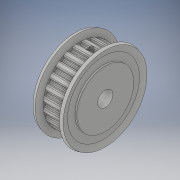
# Autodesk Inventor part: C-ATP24XL037-A-P8
Saved by Autodesk Inventor 2019 (Build 230136000, 136)
## iProperties
Created: 2023-01-11
Part Number: C-ATP24XL037-A-P8
Material: Generic
Catalog Web Link: www.cadenas.de
Description: C-ATP__XL025, C-ATP__XL031, C-ATP__ XL037, C-ATP__XL050-Economy Timing Pulleys XL Type
Vendor: MISUMI
Document SubType Name: Modeling
Designer: psAdmin
Manufacturer: MISUMI
Mass: 17.241 g
Surface Area: 69.8736 cm^2
Volume: 17.241 cm^3
Density: 1 g/cm^3
Appearance: PSOLRGB-175-175-175
Category: PARTsolutions
Company: MISUMI
Title: C-ATP24XL037-A-P8
Author: Cadenas PARTsolutions
Comments: Economy Timing Pulleys XL Type
PSOL_IDENT_0: {$CADENAS_DATA/23d-libs/misumi/metric/51_timing_pulleys/c_atp_xl.prj},239 {VTYP=3D},{NB=C-ATP24XL037
PSOL_IDENT_1: -A-P8},{LINA=C-ATP24XL037-A-P8},{NN=C-ATP__XL025, C-ATP__XL031, C-ATP__ XL037, C-ATP__XL050},{DATE=2
PSOL_IDENT_2: 2.09.2022 05:17:01},{GEOMDATE=17.04.2021 17:32:28},{VERSION=},{LINEID=110},{WBVAR=TNW,PS,SBS,DD},{WB
PSOL_IDENT_3: NUMERIC=DD}  {NB=C-ATP24XL037-A-P8},{LINA=C-ATP24XL037-A-P8},{KT=DUMMY},{PN=C-ATP24XL037-A-P8},{TYPE=
PSOL_IDENT_4: C-ATP},{MATP=},{MATPALG= 'A2017','Aluminum Alloy 2000 series','S45C','1045 Carbon Steel Equivalent','
PSOL_IDENT_5: SUS304','SUS304' },{ST=},{STALG=},{NT=24},{TNW=XL037},{TNWALG= 'XL037' },{BW=9.5mm (3/8inch)},{PS=A}
PSOL_IDENT_6: ,{PSALG= 'A' },{SBS=P},{SBSALG= 'P','Round Hole + Tap' },{DD=8.00},{DDALG=8,10},{DDHA=[8:12/1],12.7,
PSOL_IDENT_7: [13:26/1]},{DDPA=8,10},{DDNA=},{DDNK=10},{DDCA=[10,12,15,16,18,19,20]},{DDVA=[8:12/1],12.7,[13:24/1]
PSOL_IDENT_8: },{DDY=[8:24/1]},{DDWB=[8:22/1]},{DDHB=},{DDPB=},{DDNB=8,14,15},{DDCB=},{DDVFB=},{Z=0},{ZALG=[0]},{Z
PSOL_IDENT_9: MIN=10.000},{ZAMAX=26.000},{ZBMAX=0.000},{DDZ=8.000},{J=0.0},{JALG=[0]},{JMIN=2.000},{JMAX=14.0},{JP
PSOL_IDENT_10: N=},{Q=0},{QALG=[0]},{QRMIN=10.000},{QRMAX=26},{WBQMIN=12.000},{R=0},{RALG=[0]},{WBRMAX=-2.000},{S=0
PSOL_IDENT_11: .0},{SALG=[0]},{SMAX=8},{T=0.0},{TALG=[0]},{TMAX=8},{SBSPN=-P8},{A=11.0},{W=16.0},{L=0},{PD=38.81},{
PSOL_IDENT_12: OD=38.30},{D=0},{DALG=26.000},{DE=30},{F=45},{E=30},{TT=1.6},{BBK=0.000},{TTK=0.0},{ALT1=},{ALT1ALG=
PSOL_IDENT_13: '','w/o KC90 (Set Screw Angle)','KC90','with KC90 (Set Screw Angle)' },{ANG=120.000},{ALT1PN=},{ALT
PSOL_IDENT_14: 2=},{ALT2ALG= '','w/o Side Tapped Hole','QTC','with QTC (3 Places Side Tapped Hole)' },{M=},{MALG= '
PSOL_IDENT_15: N/A' },{MFTALG= 'N/A' },{MSALG= 'N/A' },{M3D=0.000},{KDML=0.000},{ML=0.000},{MUL=0.000},{PITCH=0.000
PSOL_IDENT_16: },{QSC=0.0},{QSCALG=0},{QFC=0.0},{QFCALG=0},{QTC=0.0},{QTCALG=0},{QPCDMIN=0.000},{QPCDMINALG=0.000},
PSOL_IDENT_17: {QPCDMAX=26.000},{ALT2PN=},{TAP=0.000},{ALT3=},{ALT3ALG= '','w/o Side Through Hole','KTC','with KTC
PSOL_IDENT_18: (3 Places Side Through Hole)' },{K=0.0},{KALG=0},{KMIN=4.000},{KFTMAX=7.000},{KSMAX=7.000},{KSC=0.0}
PSOL_IDENT_19: ,{KSCALG=0},{KFC=0.0},{KFCALG=0},{KTC=0.0},{KTCALG=0},{KSCMIN=12.000},{KPCDMIN=12.000},{KPCDMAX=26.0
PSOL_IDENT_20: 00},{ALT3PN=},{ALT4=},{ALT4ALG= '','w/o Side Counterbored','ZTC','with ZTC (3 Places Side Counterbor
PSOL_IDENT_21: ed)' },{ALT4MIN=18.500},{ALT4MAX=19.500},{ZM=},{ZMALG= 'N/A' },{ZMFTALG= 'N/A' },{ZMSALG= 'N/A' },{Z
PSOL_IDENT_22: MDD1=0.0},{ZMDD2=0.0},{ZMHH=0.0},{ZSC=0.0},{ZSCALG=[0]},{ZFC=0.0},{ZFCALG=[0]},{ZTC=0.0},{ZTCALG=[0]
PSOL_IDENT_23: },{ZPCDMIN=0.000},{ZPCDMINALG=0.000},{ZPCDMAX=26.000},{ALT4PN=},{ALT5=},{ALT5ALG= '','w/o Flange not
PSOL_IDENT_24: Attached','NFC','with NFC (Flange not Attached)' },{ALT5PN=},{ALT6=},{ALT6ALG= '','w/o Flange Attac
PSOL_IDENT_25: hed on One Side Only','RFC','with RFC (Flange Attached on The Boss Side Only)','LFC','with LFC (Flan
PSOL_IDENT_26: ge Attached on The Opposite Side Only)' },{ALT6PN=},{ALT7=},{ALT7ALG= '','w/o FC (Flange Cut)','FC','
PSOL_IDENT_27: with FC (Flange Cut)' },{FC=0.0},{FCALG=0},{FCMIN=39.5},{FCMAX=43.0},{ALT7PN=},{ALT8=},{ALT8ALG= '','
PSOL_IDENT_28: Not applicable' },{ALT8ALGALG=26.000},{ALT8DD2=0.000},{ALT8MM=0.000},{ALT8NN=0.000},{QC=0.000},{KC=0
PSOL_IDENT_29: .000},{ZC=0.000},{SRG=0.0},{SRGALG=[0]},{SRGMAX=0.000},{DD2=0.0},{MM=0.00},{NN=0.00},{ALT8PN=},{ALT9=
PSOL_IDENT_30: },{ALT9ALG= '','w/o BTC (Taper for Bearing Holder)','BTC','with BTC (Taper for Bearing Holder)' },{B
PSOL_IDENT_31: TC9=9.000},{TL9=1.000},{BTC=0},{BTCALG=[0]},{TL=0.0},{TLALG=0},{TLMIN=1.000},{TLMAX=-16.500},{BTCL=0
PSOL_IDENT_32: },{BTCD=0},{ALT9PN=},{WLBCTL=16.000},{ALT10=},{ALT10ALG= '','w/o TPC (Tapped Hole Dimension)','TPC','
PSOL_IDENT_33: with TPC (Tapped Hole Dimension)' },{TPC=},{TPCALG= 'N/A' },{TPCM=4.000},{ALT10PN=},{ALT11=},{ALT11A
PSOL_IDENT_34: LG= '','Not applicable' },{BC=0.0},{BCALG=0},{BCMIN=7},{BCMAX=-16.5},{M1WBC=8},{ALT11PN=},{KTT=15.15
PSOL_IDENT_35: },{ALT12=},{ALT12ALG= '','w/o SLH (Set Screw Length)','SLH','with SLH (Set Screw Length)' },{SLH=0},
PSOL_IDENT_36: {SLHALG=[0]},{ALT12PN=},{AC=M4x3},{M1=4.000},{M1L=3.000},{KEYA=1.000},{KEYB=0.000},{KEYM=1.000}
NB: C-ATP24XL037-A-P8
NN: C-ATP__XL025, C-ATP__XL031, C-ATP__ XL037, C-ATP__XL050
NT: 24
NBSYN: $PN.
LINA: C-ATP24XL037-A-P8
CATALOG: Misumi
PN: C-ATP24XL037-A-P8
TNW: XL037
PS: A
SBS: Round Hole + Tap
DD: 8
PD: 38.81
OD: 38.3
D: 0
F: 45
E: 30
SUPPLIER: MISUMI
ARTICLENO: C-ATP24XL037-A-P8
BOMINFO: C-ATP24XL037-A-P8
CREATOR: CADENAS GmbH
Autodesk Inventor part; units mm, degrees
sketch "_____2" plane through (0, 0, 0) normal (0, 0, 1) x (1, 0, 0)
  line L0 (16, 0) -> (0, 0)
  line L1 (0, 0) -> (0, 15)
  line L2 (0, 15) -> (0.9, 15)
  line L3 (0.9, 15) -> (0.9, 18.9394)
  line L4 (0.9, 18.9394) -> (0.0569, 22.0859)
  line L5 (0.0569, 22.0859) -> (1.6024, 22.5)
  line L6 (1.6024, 22.5) -> (2.5, 19.15)
  line L7 (2.5, 19.15) -> (13.5, 19.15)
  line L8 (13.5, 19.15) -> (14.3976, 22.5)
  line L9 (14.3976, 22.5) -> (15.9431, 22.0859)
  line L10 (15.9431, 22.0859) -> (15.1, 18.9394)
  line L11 (15.1, 18.9394) -> (15.1, 15)
  line L12 (15.1, 15) -> (16, 15)
  line L13 (16, 15) -> (16, 0)
  line L14 (16, 0) -> (0, 0)
  constraints: 30 end point
revolve "Revolution1" add sketch "_____2" angle 360 about axis through (16, 0, 0) along (1, 0, 0)
sketch "Sketch2" plane through (16, 0, 0) normal (1, 0, 0) x (0, 0, -1)
  point P0 (0, 0)
hole "Hole1" at (16, 0, 0) direction (-1, 0, 0) diameter 8 depth 16
sketch "_____6" plane through (2.5, 0, 0) normal (1, 0, 0) x (0, 0, -1)
  arc A0 (-19.239, 2.5329) -> (-19.239, -2.5329) centre (0, 0) ccw
  arc A1 (-19.239, -2.5329) -> (-17.9279, -7.426) centre (0, 0) ccw
  arc A2 (-17.9279, -7.426) -> (-15.395, -11.813) centre (0, 0) ccw
  arc A3 (-15.395, -11.813) -> (-11.813, -15.395) centre (0, 0) ccw
  arc A4 (-11.813, -15.395) -> (-7.426, -17.9279) centre (0, 0) ccw
  arc A5 (-7.426, -17.9279) -> (-2.5329, -19.239) centre (0, 0) ccw
  arc A6 (-2.5329, -19.239) -> (2.5329, -19.239) centre (0, 0) ccw
  arc A7 (2.5329, -19.239) -> (7.426, -17.9279) centre (0, 0) ccw
  arc A8 (7.426, -17.9279) -> (11.813, -15.395) centre (0, 0) ccw
  arc A9 (11.813, -15.395) -> (15.395, -11.813) centre (0, 0) ccw
  arc A10 (15.395, -11.813) -> (17.9279, -7.426) centre (0, 0) ccw
  arc A11 (17.9279, -7.426) -> (19.239, -2.5329) centre (0, 0) ccw
  arc A12 (19.239, -2.5329) -> (19.239, 2.5329) centre (0, 0) ccw
  arc A13 (19.239, 2.5329) -> (17.9279, 7.426) centre (0, 0) ccw
  arc A14 (17.9279, 7.426) -> (15.395, 11.813) centre (0, 0) ccw
  arc A15 (15.395, 11.813) -> (11.813, 15.395) centre (0, 0) ccw
  arc A16 (11.813, 15.395) -> (7.426, 17.9279) centre (0, 0) ccw
  arc A17 (7.426, 17.9279) -> (2.5329, 19.239) centre (0, 0) ccw
  arc A18 (2.5329, 19.239) -> (-2.5329, 19.239) centre (0, 0) ccw
  arc A19 (-2.5329, 19.239) -> (-7.426, 17.9279) centre (0, 0) ccw
  arc A20 (-7.426, 17.9279) -> (-11.813, 15.395) centre (0, 0) ccw
  arc A21 (-11.813, 15.395) -> (-15.395, 11.813) centre (0, 0) ccw
  arc A22 (-15.395, 11.813) -> (-17.9279, 7.426) centre (0, 0) ccw
  arc A23 (-17.9279, 7.426) -> (-19.239, 2.5329) centre (0, 0) ccw
  arc A24 (-18.7244, -1.0947) -> (-19.0742, -1.7017) centre (-18.4667, -1.6475) ccw
  arc A25 (-19.0742, -1.7017) -> (-18.9862, -2.4996) centre (0, 0) ccw
  arc A26 (-18.9862, -2.4996) -> (-18.8647, -3.293) centre (0, 0) ccw
  arc A27 (-18.8647, -3.293) -> (-18.3698, -3.7889) centre (-18.2638, -3.1881) ccw
  line L0 (-18.3698, -3.7889) -> (-17.6918, -3.9084)
  arc A28 (-17.2064, -4.3593) -> (-17.6918, -3.9084) centre (-17.7977, -4.5091) ccw
  arc A29 (-17.2064, -4.3593) -> (-17.0808, -4.8279) centre (0, 0) ccw
  arc A30 (-17.2757, -5.4611) -> (-17.0808, -4.8279) centre (-17.6678, -4.9938) ccw
  line L1 (-17.2757, -5.4611) -> (-17.8031, -5.9036)
  arc A31 (-17.8031, -5.9036) -> (-17.9839, -6.5805) centre (-17.411, -6.3709) ccw
  arc A32 (-17.9839, -6.5805) -> (-17.6923, -7.3284) centre (0, 0) ccw
  arc A33 (-17.6923, -7.3284) -> (-17.3696, -8.0634) centre (0, 0) ccw
  arc A34 (-17.3696, -8.0634) -> (-16.7632, -8.4142) centre (-16.8164, -7.8065) ccw
  line L2 (-16.7632, -8.4142) -> (-16.0773, -8.3542)
  arc A35 (-15.4918, -8.6641) -> (-16.0773, -8.3542) centre (-16.0242, -8.9619) ccw
  arc A36 (-15.4918, -8.6641) -> (-15.2492, -9.0842) centre (0, 0) ccw
  arc A37 (-15.2736, -9.7463) -> (-15.2492, -9.0842) centre (-15.7733, -9.3964) ccw
  line L3 (-15.2736, -9.7463) -> (-15.6685, -10.3103)
  arc A38 (-15.6685, -10.3103) -> (-15.6679, -11.0109) centre (-15.1688, -10.6601) ccw
  arc A39 (-15.6679, -11.0109) -> (-15.1927, -11.6578) centre (0, 0) ccw
  arc A40 (-15.1927, -11.6578) -> (-14.6908, -12.2842) centre (0, 0) ccw
  arc A41 (-14.6908, -12.2842) -> (-14.0142, -12.4661) centre (-14.2229, -11.8929) ccw
  line L4 (-14.0142, -12.4661) -> (-13.3673, -12.2307)
  arc A42 (-12.7215, -12.3785) -> (-13.3673, -12.2307) centre (-13.1587, -12.8039) ccw
  arc A43 (-12.7215, -12.3785) -> (-12.3785, -12.7215) centre (0, 0) ccw
  arc A44 (-12.2307, -13.3673) -> (-12.3785, -12.7215) centre (-12.8039, -13.1587) ccw
  line L5 (-12.2307, -13.3673) -> (-12.4661, -14.0142)
  arc A45 (-12.4661, -14.0142) -> (-12.2842, -14.6908) centre (-11.8929, -14.2229) ccw
  arc A46 (-12.2842, -14.6908) -> (-11.6578, -15.1927) centre (0, 0) ccw
  arc A47 (-11.6578, -15.1927) -> (-11.0109, -15.6679) centre (0, 0) ccw
  arc A48 (-11.0109, -15.6679) -> (-10.3103, -15.6685) centre (-10.6601, -15.1688) ccw
  line L6 (-10.3103, -15.6685) -> (-9.7463, -15.2736)
  arc A49 (-9.0842, -15.2492) -> (-9.7463, -15.2736) centre (-9.3964, -15.7733) ccw
  arc A50 (-9.0842, -15.2492) -> (-8.6641, -15.4918) centre (0, 0) ccw
  arc A51 (-8.3542, -16.0773) -> (-8.6641, -15.4918) centre (-8.9619, -16.0242) ccw
  line L7 (-8.3542, -16.0773) -> (-8.4142, -16.7632)
  arc A52 (-8.4142, -16.7632) -> (-8.0634, -17.3696) centre (-7.8065, -16.8164) ccw
  arc A53 (-8.0634, -17.3696) -> (-7.3284, -17.6923) centre (0, 0) ccw
  arc A54 (-7.3284, -17.6923) -> (-6.5805, -17.9839) centre (0, 0) ccw
  arc A55 (-6.5805, -17.9839) -> (-5.9036, -17.8031) centre (-6.3709, -17.411) ccw
  line L8 (-5.9036, -17.8031) -> (-5.4611, -17.2757)
  arc A56 (-4.8279, -17.0808) -> (-5.4611, -17.2757) centre (-4.9938, -17.6678) ccw
  arc A57 (-4.8279, -17.0808) -> (-4.3593, -17.2064) centre (0, 0) ccw
  arc A58 (-3.9084, -17.6918) -> (-4.3593, -17.2064) centre (-4.5091, -17.7977) ccw
  line L9 (-3.9084, -17.6918) -> (-3.7889, -18.3698)
  arc A59 (-3.7889, -18.3698) -> (-3.293, -18.8647) centre (-3.1881, -18.2638) ccw
  arc A60 (-3.293, -18.8647) -> (-2.4996, -18.9862) centre (0, 0) ccw
  arc A61 (-2.4996, -18.9862) -> (-1.7017, -19.0742) centre (0, 0) ccw
  arc A62 (-1.7017, -19.0742) -> (-1.0947, -18.7244) centre (-1.6475, -18.4667) ccw
  line L10 (-1.0947, -18.7244) -> (-0.8037, -18.1005)
  arc A63 (-0.2426, -17.7483) -> (-0.8037, -18.1005) centre (-0.2509, -18.3583) ccw
  arc A64 (-0.2426, -17.7483) -> (0.2426, -17.7483) centre (0, 0) ccw
  arc A65 (0.8037, -18.1005) -> (0.2426, -17.7483) centre (0.2509, -18.3583) ccw
  line L11 (0.8037, -18.1005) -> (1.0947, -18.7244)
  arc A66 (1.0947, -18.7244) -> (1.7017, -19.0742) centre (1.6475, -18.4667) ccw
  arc A67 (1.7017, -19.0742) -> (2.4996, -18.9862) centre (0, 0) ccw
  arc A68 (2.4996, -18.9862) -> (3.293, -18.8647) centre (0, 0) ccw
  arc A69 (3.293, -18.8647) -> (3.7889, -18.3698) centre (3.1881, -18.2638) ccw
  line L12 (3.7889, -18.3698) -> (3.9084, -17.6918)
  arc A70 (4.3593, -17.2064) -> (3.9084, -17.6918) centre (4.5091, -17.7977) ccw
  arc A71 (4.3593, -17.2064) -> (4.8279, -17.0808) centre (0, 0) ccw
  arc A72 (5.4611, -17.2757) -> (4.8279, -17.0808) centre (4.9938, -17.6678) ccw
  line L13 (5.4611, -17.2757) -> (5.9036, -17.8031)
  arc A73 (5.9036, -17.8031) -> (6.5805, -17.9839) centre (6.3709, -17.411) ccw
  arc A74 (6.5805, -17.9839) -> (7.3284, -17.6923) centre (0, 0) ccw
  arc A75 (7.3284, -17.6923) -> (8.0634, -17.3696) centre (0, 0) ccw
  arc A76 (8.0634, -17.3696) -> (8.4142, -16.7632) centre (7.8065, -16.8164) ccw
  line L14 (8.4142, -16.7632) -> (8.3542, -16.0773)
  arc A77 (8.6641, -15.4918) -> (8.3542, -16.0773) centre (8.9619, -16.0242) ccw
  arc A78 (8.6641, -15.4918) -> (9.0842, -15.2492) centre (0, 0) ccw
  arc A79 (9.7463, -15.2736) -> (9.0842, -15.2492) centre (9.3964, -15.7733) ccw
  line L15 (9.7463, -15.2736) -> (10.3103, -15.6685)
  arc A80 (10.3103, -15.6685) -> (11.0109, -15.6679) centre (10.6601, -15.1688) ccw
  arc A81 (11.0109, -15.6679) -> (11.6578, -15.1927) centre (0, 0) ccw
  arc A82 (11.6578, -15.1927) -> (12.2842, -14.6908) centre (0, 0) ccw
  arc A83 (12.2842, -14.6908) -> (12.4661, -14.0142) centre (11.8929, -14.2229) ccw
  line L16 (12.4661, -14.0142) -> (12.2307, -13.3673)
  arc A84 (12.3785, -12.7215) -> (12.2307, -13.3673) centre (12.8039, -13.1587) ccw
  arc A85 (12.3785, -12.7215) -> (12.7215, -12.3785) centre (0, 0) ccw
  arc A86 (13.3673, -12.2307) -> (12.7215, -12.3785) centre (13.1587, -12.8039) ccw
  line L17 (13.3673, -12.2307) -> (14.0142, -12.4661)
  arc A87 (14.0142, -12.4661) -> (14.6908, -12.2842) centre (14.2229, -11.8929) ccw
  arc A88 (14.6908, -12.2842) -> (15.1927, -11.6578) centre (0, 0) ccw
  arc A89 (15.1927, -11.6578) -> (15.6679, -11.0109) centre (0, 0) ccw
  arc A90 (15.6679, -11.0109) -> (15.6685, -10.3103) centre (15.1688, -10.6601) ccw
  line L18 (15.6685, -10.3103) -> (15.2736, -9.7463)
  arc A91 (15.2492, -9.0842) -> (15.2736, -9.7463) centre (15.7733, -9.3964) ccw
  arc A92 (15.2492, -9.0842) -> (15.4918, -8.6641) centre (0, 0) ccw
  arc A93 (16.0773, -8.3542) -> (15.4918, -8.6641) centre (16.0242, -8.9619) ccw
  line L19 (16.0773, -8.3542) -> (16.7632, -8.4142)
  arc A94 (16.7632, -8.4142) -> (17.3696, -8.0634) centre (16.8164, -7.8065) ccw
  arc A95 (17.3696, -8.0634) -> (17.6923, -7.3284) centre (0, 0) ccw
  arc A96 (17.6923, -7.3284) -> (17.9839, -6.5805) centre (0, 0) ccw
  arc A97 (17.9839, -6.5805) -> (17.8031, -5.9036) centre (17.411, -6.3709) ccw
  line L20 (17.8031, -5.9036) -> (17.2757, -5.4611)
  arc A98 (17.0808, -4.8279) -> (17.2757, -5.4611) centre (17.6678, -4.9938) ccw
  arc A99 (17.0808, -4.8279) -> (17.2064, -4.3593) centre (0, 0) ccw
  arc A100 (17.6918, -3.9084) -> (17.2064, -4.3593) centre (17.7977, -4.5091) ccw
  line L21 (17.6918, -3.9084) -> (18.3698, -3.7889)
  arc A101 (18.3698, -3.7889) -> (18.8647, -3.293) centre (18.2638, -3.1881) ccw
  arc A102 (18.8647, -3.293) -> (18.9862, -2.4996) centre (0, 0) ccw
  arc A103 (18.9862, -2.4996) -> (19.0742, -1.7017) centre (0, 0) ccw
  arc A104 (19.0742, -1.7017) -> (18.7244, -1.0947) centre (18.4667, -1.6475) ccw
  line L22 (18.7244, -1.0947) -> (18.1005, -0.8037)
  arc A105 (17.7483, -0.2426) -> (18.1005, -0.8037) centre (18.3583, -0.2509) ccw
  arc A106 (17.7483, -0.2426) -> (17.7483, 0.2426) centre (0, 0) ccw
  arc A107 (18.1005, 0.8037) -> (17.7483, 0.2426) centre (18.3583, 0.2509) ccw
  line L23 (18.1005, 0.8037) -> (18.7244, 1.0947)
  arc A108 (18.7244, 1.0947) -> (19.0742, 1.7017) centre (18.4667, 1.6475) ccw
  arc A109 (19.0742, 1.7017) -> (18.9862, 2.4996) centre (0, 0) ccw
  arc A110 (18.9862, 2.4996) -> (18.8647, 3.293) centre (0, 0) ccw
  arc A111 (18.8647, 3.293) -> (18.3698, 3.7889) centre (18.2638, 3.1881) ccw
  line L24 (18.3698, 3.7889) -> (17.6918, 3.9084)
  arc A112 (17.2064, 4.3593) -> (17.6918, 3.9084) centre (17.7977, 4.5091) ccw
  arc A113 (17.2064, 4.3593) -> (17.0808, 4.8279) centre (0, 0) ccw
  arc A114 (17.2757, 5.4611) -> (17.0808, 4.8279) centre (17.6678, 4.9938) ccw
  line L25 (17.2757, 5.4611) -> (17.8031, 5.9036)
  arc A115 (17.8031, 5.9036) -> (17.9839, 6.5805) centre (17.411, 6.3709) ccw
  arc A116 (17.9839, 6.5805) -> (17.6923, 7.3284) centre (0, 0) ccw
  arc A117 (17.6923, 7.3284) -> (17.3696, 8.0634) centre (0, 0) ccw
  arc A118 (17.3696, 8.0634) -> (16.7632, 8.4142) centre (16.8164, 7.8065) ccw
  line L26 (16.7632, 8.4142) -> (16.0773, 8.3542)
  arc A119 (15.4918, 8.6641) -> (16.0773, 8.3542) centre (16.0242, 8.9619) ccw
  arc A120 (15.4918, 8.6641) -> (15.2492, 9.0842) centre (0, 0) ccw
  arc A121 (15.2736, 9.7463) -> (15.2492, 9.0842) centre (15.7733, 9.3964) ccw
  line L27 (15.2736, 9.7463) -> (15.6685, 10.3103)
  arc A122 (15.6685, 10.3103) -> (15.6679, 11.0109) centre (15.1688, 10.6601) ccw
  arc A123 (15.6679, 11.0109) -> (15.1927, 11.6578) centre (0, 0) ccw
  arc A124 (15.1927, 11.6578) -> (14.6908, 12.2842) centre (0, 0) ccw
  arc A125 (14.6908, 12.2842) -> (14.0142, 12.4661) centre (14.2229, 11.8929) ccw
  line L28 (14.0142, 12.4661) -> (13.3673, 12.2307)
  arc A126 (12.7215, 12.3785) -> (13.3673, 12.2307) centre (13.1587, 12.8039) ccw
  arc A127 (12.7215, 12.3785) -> (12.3785, 12.7215) centre (0, 0) ccw
  arc A128 (12.2307, 13.3673) -> (12.3785, 12.7215) centre (12.8039, 13.1587) ccw
  line L29 (12.2307, 13.3673) -> (12.4661, 14.0142)
  arc A129 (12.4661, 14.0142) -> (12.2842, 14.6908) centre (11.8929, 14.2229) ccw
  arc A130 (12.2842, 14.6908) -> (11.6578, 15.1927) centre (0, 0) ccw
  arc A131 (11.6578, 15.1927) -> (11.0109, 15.6679) centre (0, 0) ccw
  arc A132 (11.0109, 15.6679) -> (10.3103, 15.6685) centre (10.6601, 15.1688) ccw
  line L30 (10.3103, 15.6685) -> (9.7463, 15.2736)
  arc A133 (9.0842, 15.2492) -> (9.7463, 15.2736) centre (9.3964, 15.7733) ccw
  arc A134 (9.0842, 15.2492) -> (8.6641, 15.4918) centre (0, 0) ccw
  arc A135 (8.3542, 16.0773) -> (8.6641, 15.4918) centre (8.9619, 16.0242) ccw
  line L31 (8.3542, 16.0773) -> (8.4142, 16.7632)
  arc A136 (8.4142, 16.7632) -> (8.0634, 17.3696) centre (7.8065, 16.8164) ccw
  arc A137 (8.0634, 17.3696) -> (7.3284, 17.6923) centre (0, 0) ccw
  arc A138 (7.3284, 17.6923) -> (6.5805, 17.9839) centre (0, 0) ccw
  arc A139 (6.5805, 17.9839) -> (5.9036, 17.8031) centre (6.3709, 17.411) ccw
  line L32 (5.9036, 17.8031) -> (5.4611, 17.2757)
  arc A140 (4.8279, 17.0808) -> (5.4611, 17.2757) centre (4.9938, 17.6678) ccw
  arc A141 (4.8279, 17.0808) -> (4.3593, 17.2064) centre (0, 0) ccw
  arc A142 (3.9084, 17.6918) -> (4.3593, 17.2064) centre (4.5091, 17.7977) ccw
  line L33 (3.9084, 17.6918) -> (3.7889, 18.3698)
  arc A143 (3.7889, 18.3698) -> (3.293, 18.8647) centre (3.1881, 18.2638) ccw
  arc A144 (3.293, 18.8647) -> (2.4996, 18.9862) centre (0, 0) ccw
  arc A145 (2.4996, 18.9862) -> (1.7017, 19.0742) centre (0, 0) ccw
  arc A146 (1.7017, 19.0742) -> (1.0947, 18.7244) centre (1.6475, 18.4667) ccw
  line L34 (1.0947, 18.7244) -> (0.8037, 18.1005)
  arc A147 (0.2426, 17.7483) -> (0.8037, 18.1005) centre (0.2509, 18.3583) ccw
  arc A148 (0.2426, 17.7483) -> (-0.2426, 17.7483) centre (0, 0) ccw
  arc A149 (-0.8037, 18.1005) -> (-0.2426, 17.7483) centre (-0.2509, 18.3583) ccw
  line L35 (-0.8037, 18.1005) -> (-1.0947, 18.7244)
  arc A150 (-1.0947, 18.7244) -> (-1.7017, 19.0742) centre (-1.6475, 18.4667) ccw
  arc A151 (-1.7017, 19.0742) -> (-2.4996, 18.9862) centre (0, 0) ccw
  arc A152 (-2.4996, 18.9862) -> (-3.293, 18.8647) centre (0, 0) ccw
  arc A153 (-3.293, 18.8647) -> (-3.7889, 18.3698) centre (-3.1881, 18.2638) ccw
  line L36 (-3.7889, 18.3698) -> (-3.9084, 17.6918)
  arc A154 (-4.3593, 17.2064) -> (-3.9084, 17.6918) centre (-4.5091, 17.7977) ccw
  arc A155 (-4.3593, 17.2064) -> (-4.8279, 17.0808) centre (0, 0) ccw
  arc A156 (-5.4611, 17.2757) -> (-4.8279, 17.0808) centre (-4.9938, 17.6678) ccw
  line L37 (-5.4611, 17.2757) -> (-5.9036, 17.8031)
  arc A157 (-5.9036, 17.8031) -> (-6.5805, 17.9839) centre (-6.3709, 17.411) ccw
  arc A158 (-6.5805, 17.9839) -> (-7.3284, 17.6923) centre (0, 0) ccw
  arc A159 (-7.3284, 17.6923) -> (-8.0634, 17.3696) centre (0, 0) ccw
  arc A160 (-8.0634, 17.3696) -> (-8.4142, 16.7632) centre (-7.8065, 16.8164) ccw
  line L38 (-8.4142, 16.7632) -> (-8.3542, 16.0773)
  arc A161 (-8.6641, 15.4918) -> (-8.3542, 16.0773) centre (-8.9619, 16.0242) ccw
  arc A162 (-8.6641, 15.4918) -> (-9.0842, 15.2492) centre (0, 0) ccw
  arc A163 (-9.7463, 15.2736) -> (-9.0842, 15.2492) centre (-9.3964, 15.7733) ccw
  line L39 (-9.7463, 15.2736) -> (-10.3103, 15.6685)
  arc A164 (-10.3103, 15.6685) -> (-11.0109, 15.6679) centre (-10.6601, 15.1688) ccw
  arc A165 (-11.0109, 15.6679) -> (-11.6578, 15.1927) centre (0, 0) ccw
  arc A166 (-11.6578, 15.1927) -> (-12.2842, 14.6908) centre (0, 0) ccw
  arc A167 (-12.2842, 14.6908) -> (-12.4661, 14.0142) centre (-11.8929, 14.2229) ccw
  line L40 (-12.4661, 14.0142) -> (-12.2307, 13.3673)
  arc A168 (-12.3785, 12.7215) -> (-12.2307, 13.3673) centre (-12.8039, 13.1587) ccw
  arc A169 (-12.3785, 12.7215) -> (-12.7215, 12.3785) centre (0, 0) ccw
  arc A170 (-13.3673, 12.2307) -> (-12.7215, 12.3785) centre (-13.1587, 12.8039) ccw
  line L41 (-13.3673, 12.2307) -> (-14.0142, 12.4661)
  arc A171 (-14.0142, 12.4661) -> (-14.6908, 12.2842) centre (-14.2229, 11.8929) ccw
  arc A172 (-14.6908, 12.2842) -> (-15.1927, 11.6578) centre (0, 0) ccw
  arc A173 (-15.1927, 11.6578) -> (-15.6679, 11.0109) centre (0, 0) ccw
  arc A174 (-15.6679, 11.0109) -> (-15.6685, 10.3103) centre (-15.1688, 10.6601) ccw
  line L42 (-15.6685, 10.3103) -> (-15.2736, 9.7463)
  arc A175 (-15.2492, 9.0842) -> (-15.2736, 9.7463) centre (-15.7733, 9.3964) ccw
  arc A176 (-15.2492, 9.0842) -> (-15.4918, 8.6641) centre (0, 0) ccw
  arc A177 (-16.0773, 8.3542) -> (-15.4918, 8.6641) centre (-16.0242, 8.9619) ccw
  line L43 (-16.0773, 8.3542) -> (-16.7632, 8.4142)
  arc A178 (-16.7632, 8.4142) -> (-17.3696, 8.0634) centre (-16.8164, 7.8065) ccw
  arc A179 (-17.3696, 8.0634) -> (-17.6923, 7.3284) centre (0, 0) ccw
  arc A180 (-17.6923, 7.3284) -> (-17.9839, 6.5805) centre (0, 0) ccw
  arc A181 (-17.9839, 6.5805) -> (-17.8031, 5.9036) centre (-17.411, 6.3709) ccw
  line L44 (-17.8031, 5.9036) -> (-17.2757, 5.4611)
  arc A182 (-17.0808, 4.8279) -> (-17.2757, 5.4611) centre (-17.6678, 4.9938) ccw
  arc A183 (-17.0808, 4.8279) -> (-17.2064, 4.3593) centre (0, 0) ccw
  arc A184 (-17.6918, 3.9084) -> (-17.2064, 4.3593) centre (-17.7977, 4.5091) ccw
  line L45 (-17.6918, 3.9084) -> (-18.3698, 3.7889)
  arc A185 (-18.3698, 3.7889) -> (-18.8647, 3.293) centre (-18.2638, 3.1881) ccw
  arc A186 (-18.8647, 3.293) -> (-18.9862, 2.4996) centre (0, 0) ccw
  arc A187 (-18.9862, 2.4996) -> (-19.0742, 1.7017) centre (0, 0) ccw
  arc A188 (-19.0742, 1.7017) -> (-18.7244, 1.0947) centre (-18.4667, 1.6475) ccw
  line L46 (-18.7244, 1.0947) -> (-18.1005, 0.8037)
  arc A189 (-17.7483, 0.2426) -> (-18.1005, 0.8037) centre (-18.3583, 0.2509) ccw
  arc A190 (-17.7483, 0.2426) -> (-17.7483, -0.2426) centre (0, 0) ccw
  arc A191 (-18.1005, -0.8037) -> (-17.7483, -0.2426) centre (-18.3583, -0.2509) ccw
  line L47 (-18.1005, -0.8037) -> (-18.7244, -1.0947)
  constraints: 384 point on circle, 192 centre point, 96 end point
extrude "Extrusion1" cut sketch "_____6" along normal blind 11
sketch "_____15" plane through (8, 0, 0) normal (1, 0, 0) x (0, 0, -1)
  line L0 (0, 0) -> (0, 19.15)
  line L1 (0, 19.15) -> (1.621, 19.15)
  line L2 (1.621, 19.15) -> (1.621, 0)
  line L3 (1.621, 0) -> (0, 0)
  line L4 (0, 0) -> (0, 19.15)
  constraints: 10 end point
revolve "Revolution2" cut sketch "_____15" angle 360 about axis through (8, 0, 0) along (0, -1, 0)
thread "Thread1" size "M4x0.7" class "6H" standard "ISO Metric profile" length 15.15
sketch "_____16" plane through (8, 0, 0) normal (1, 0, 0) x (0, 0, -1)
  line L0 (0, 0) -> (16.5844, -9.575)
  line L1 (16.5844, -9.575) -> (15.7739, -10.9788)
  line L2 (15.7739, -10.9788) -> (-0.8105, -1.4038)
  line L3 (-0.8105, -1.4038) -> (0, 0)
  line L4 (0, 0) -> (16.5844, -9.575)
  constraints: 10 end point
revolve "Revolution3" cut sketch "_____16" angle 360 about axis through (8, 0, 0) along (0, 0.5, 0.8660254)
thread "Thread2" size "M4x0.7" class "6H" standard "ISO Metric profile" length 15.15
ref_plane "to_screw1_XY" through (8, 4, 0) normal (0, 1, 0) x (1, 0, 0)
ref_plane "to_screw1_YZ" through (8, 4, 0) normal (1, 0, 0) x (0, 0, -1)
ref_plane "to_screw1_ZX" through (8, 4, 0) normal (0, 0, -1) x (0, 1, 0)
ref_plane "to_screw2_XY" through (8, -2, -3.4641) normal (0, -0.5, -0.8660254) x (1, 0, 0)
ref_plane "to_screw2_YZ" through (8, -2, -3.4641) normal (1, 0, 0) x (0, -0.8660254, 0.5)
ref_plane "to_screw2_ZX" through (8, -2, -3.4641) normal (0, -0.8660254, 0.5) x (0, -0.5, -0.8660254)
body "Solid1"
